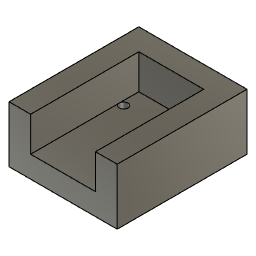
DrzacPrijemnikIRSenzora v3 (Autodesk Fusion 360 design; units mm, degrees)
Autodesk Fusion 360 part; units mm, degrees
sketch "Sketch1" plane through (0, 0, 0) normal (0, 0, 1) x (1, 0, 0)
  line L0 (50, 50) -> (65, 50)
  line L1 (65, 50) -> (65, 31)
  line L2 (50, 31) -> (50, 50)
  line L3 (45, 55) -> (70, 55)
  line L4 (70, 55) -> (70, 25)
  line L5 (70, 25) -> (45, 25)
  line L6 (45, 25) -> (45, 55)
  line L7 (50, 31) -> (50, 25)
  line L8 (65, 31) -> (65, 25)
  line L9 (50, 50) -> (50, 48.5)
  line L10 (50, 50) -> (50, 48)
  circle A0 centre (52.5, 48) radius 1.25
  line L11 (65, 50) -> (65, 48)
  circle A1 centre (62.5, 48) radius 1.25
  dimension "d1" = 15
  dimension "d2" = 19
  dimension "d4" = 2
  dimension "d5" = 2.5
  dimension "d6" = 2.5
  dimension "d7" = 2
  dimension "d8" = 2.5
  dimension "d9" = 2.5
  constraint horizontal L0
  constraint vertical L1
  constraint vertical L2
  constraint horizontal L3
  constraint vertical L4
  constraint horizontal L5
  constraint vertical L6
  constraint perpendicular L5 L7
  constraint coincident L5 L8.end
  constraint perpendicular L5 L8
  constraint coincident L2 L9.end
  constraint perpendicular L0 L10
  constraint perpendicular L0 L11
  measures "d1" distance of L0.start L0.end
  measures "d2" distance of L0.start L2.start
  measures "d4" distance of L0.start L10.end
  measures "d5" distance of L10.end A0.centre
  measures "d6" diameter of A0
  measures "d7" distance of L0.end L11.end
  measures "d8" distance of L11.end A1.centre
  measures "d9" diameter of A1
extrude "Extrude1" add sketch "Sketch1" along normal blind 8 contours L0 L1 L2 L3 L4 L5 L6 L7 L8 L9 L10 L11
extrude "Extrude2" add 1 faces at (46.6667, 42.6667, 8) along direction (0, 0, 1) blind 5
sketch "Sketch2" plane through (0, 0, 13) normal (0, 0, 1) x (-1, 0, 0)
  line L0 (-50, -50) -> (-65, -50)
  line L1 (-65, -50) -> (-65, -25)
  line L2 (-65, -25) -> (-70, -25)
  line L3 (-70, -25) -> (-70, -55)
  line L4 (-70, -55) -> (-45, -55)
  line L5 (-45, -55) -> (-45, -25)
  line L6 (-45, -25) -> (-50, -25)
  line L7 (-50, -25) -> (-50, -50)
  line L8 (-50, -25) -> (-65, -25)
  constraint coincident L6.end L7.start
  constraint coincident L1.end L2.start
extrude "Extrude3" add sketch "Sketch2" against normal blind 5 contours L0 L1 L7 L8
move_body "Move1" bodies 1 to x (-1, 0, 0) y (0, 1, 0) z (0, 0, -1) at (115, 0, 16)
sketch "Sketch3" plane through (0, 0, 8) normal (0, 0, 1) x (-1, 0, 0)
  line L0 (-65, -25) -> (-65, -50)
  line L1 (-65, -50) -> (-50, -50)
  line L2 (-50, -50) -> (-50, -25)
  line L3 (-50, -25) -> (-65, -25)
  line L4 (-50, -50) -> (-50, -45.5)
  line L5 (-50, -45.5) -> (-51, -45.5)
  circle A0 centre (-51, -45.5) radius 1
  line L6 (-65, -50) -> (-65, -45.5)
  line L7 (-65, -45.5) -> (-64, -45.5)
  circle A1 centre (-64, -45.5) radius 1
  dimension "d16" = 4.5
  dimension "d17" = 1
  dimension "d18" = 2
  dimension "d19" = 4.5
  dimension "d20" = 1
  dimension "d21" = 2
  constraint coincident L1.end L2.start
  constraint perpendicular L1 L4
  constraint perpendicular L4 L5
  constraint coincident L5.end A0.centre
  constraint coincident L0.end L1.start
  constraint perpendicular L1 L6
  constraint perpendicular L6 L7
  constraint coincident L7.end A1.centre
  measures "d16" distance of L1.end L4.end
  measures "d17" distance of L4.end L5.end
  measures "d18" diameter of A0
  measures "d19" distance of L0.end L6.end
  measures "d20" distance of L6.end L7.end
  measures "d21" diameter of A1
extrude "Extrude4" cut sketch "Sketch3" against normal blind 50 contours A1 | A0
extrude "Extrude5" cut 1 faces at (65, 40.1667, 13.3333) along direction (1, 0, 0) blind 3
extrude "Extrude6" add 1 faces at (70, 35, 11.6667) along direction (1, 0, 0) blind 3
extrude "Extrude7" cut 1 faces at (50, 40.1667, 13.3333) along direction (-1, 0, 0) blind 3
extrude "Extrude8" add 1 faces at (45, 45, 11.6667) along direction (-1, 0, 0) blind 3
extrude "Extrude9" add 1 faces at (47, 41.6667, 13.3333) along direction (1, 0, 0) blind 3
extrude "Extrude10" cut 1 faces at (42, 45, 11.6667) along direction (1, 0, 0) blind 3
extrude "Extrude11" add 1 faces at (68, 33.3333, 13.3333) along direction (-1, 0, 0) blind 3
extrude "Extrude12" cut 1 faces at (73, 35, 11.6667) along direction (-1, 0, 0) blind 3
